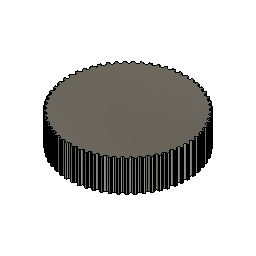
gear_61z (Autodesk Fusion 360 design; units mm, degrees)
Autodesk Fusion 360 part; units mm, degrees
sketch "Sketch1" plane through (0, 0, 0) normal (0, 0, 1) x (1, 0, 0) in component "gt2 pulley"
  circle A0 centre (0, 0) radius 19.4169 construction
  circle A1 centre (0, 0) radius 18.4129 construction
  line L0 (0, 0) -> (0, 19.4169) construction
  line L1 (0, 0) -> (0.9996, 19.3912) construction
  line L2 (0, 0) -> (1.4062, 19.3659) construction
  circle A2 centre (0, 0) radius 19.1629 construction
  arc A3 (0.3916, 19.0246) -> (0.4635, 18.7309) centre (1.3878, 19.1126) ccw
  circle A4 centre (0, 0) radius 19.0129 construction
  arc A5 (0.2441, 19.1613) -> (0, 19.1629) centre (0, 0) ccw
  arc A6 (0.3916, 19.0246) -> (0.2441, 19.1613) centre (0.2422, 19.0114) ccw
  arc A7 (0.4635, 18.7309) -> (0.9479, 18.3885) centre (0.9764, 18.9428) ccw
  arc A8 (0, 19.1629) -> (-0.2441, 19.1613) centre (0, 0) ccw
  arc A9 (-0.2441, 19.1613) -> (-0.3916, 19.0246) centre (-0.2422, 19.0114) ccw
  arc A10 (-0.4635, 18.7309) -> (-0.3916, 19.0246) centre (-1.3878, 19.1126) ccw
  arc A11 (-0.9479, 18.3885) -> (-0.4635, 18.7309) centre (-0.9764, 18.9427) ccw
  arc A12 (0.9479, 18.3885) -> (-0.9479, 18.3885) centre (0, 0) ccw
  point P0 (1.3878, 19.1126)
  point P1 (0, 19.1629)
  dimension "d18" = 38.8338
  dimension "d19" = 2.951
  dimension "d22" = 1.004
  dimension "d24" = 0.75
  dimension "d26" = 1
  dimension "d27" = 0.15
  dimension "d28" = 0.15
  dimension "d47" = 0.555
  dimension "d52" = 3.812
  constraint coincident A0.centre A1.centre
  constraint coincident A0 L0.end
  constraint vertical L0
  constraint coincident A0 L1.end
  constraint coincident A0 L2.end
  constraint concentric A1 A2
  constraint coincident A1 A7.end
  constraint coincident L1 A7.end
  constraint coincident A2 P0
  constraint coincident L2 P0
  constraint coincident P0 A3.centre
  constraint coincident A2 P1
  constraint coincident L0 P1
  constraint concentric A2 A4
  constraint coincident P1 A5.end
  constraint coincident A4 A6.centre
  constraint coincident A3.start A6.start
  constraint tangent A3 A6
  constraint tangent A3 A7
  constraint symmetric L0 A7.end A11.start
  constraint symmetric L0 A3.start A9.end
  constraint symmetric L0 A3.end A10.start
  constraint symmetric L0 A3 A10
  constraint symmetric L0 A5.start A8.end
  constraint symmetric L0 P1 A5.end
  constraint symmetric L0 A5 A8
  constraint symmetric L0 A6 A9
  constraint symmetric L0 A7 A11
  constraint coincident A1 A11.start
  constraint tangent A1 A7
  constraint coincident L1 A7.centre
  measures "d18" diameter of A0
  measures "d19" angle of L0 L1
  measures "d22" distance of A0 A1
  measures "d24" distance of A1 A2
  measures "d26" radius of A3
  measures "d27" distance of A2 A4
  measures "d28" radius of A6
  measures "d47" radius of A7
extrude "Extrude1" add sketch "Sketch1" along normal blind 10 makes body 1
pattern_circular "C-Pattern1" count 61 over 360 about axis through (0, 0, 1.75) along (0, 0, 1) of bodies 1 makes body 2 at (-2.6252, 18.2248, 6.6667) makes body 3 at (-3.8695, 18.0017, 6.6667) makes body 4 at (-6.2976, 17.3025, 6.6667) makes body 5 at (-6.6919, 17.1538, 3.3333) makes body 6 at (-9.1608, 15.9723, 6.6667) makes body 7 at (-10.0593, 15.4222, 3.3333) makes body 8 at (-12.6994, 13.3327, 6.6667) makes body 9 at (-13.0012, 13.0385, 6.6667) makes body 10 at (-14.273, 11.6326, 3.3333) makes body 11 at (-15.3934, 10.1034, 3.3333) makes body 12 at (-16.9758, 7.1314, 6.6667) makes body 13 at (-17.1346, 6.741, 3.3333) makes body 14 at (-17.7369, 4.9435, 3.3333) makes body 15 at (-18.2737, 2.2597, 6.6667) makes body 16 at (-18.411, -0.2634, 6.6667) makes body 17 at (-18.4002, -0.6847, 3.3333) makes body 18 at (-18.2322, -2.573, 3.3333) makes body 19 at (-17.4589, -5.85, 6.6667) makes body 20 at (-17.0163, -7.0341, 6.6667) makes body 21 at (-16.2029, -8.7465, 6.6667) makes body 22 at (-15.6761, -9.6589, 3.3333) makes body 23 at (-14.0712, -11.8759, 6.6667) makes body 24 at (-13.3689, -12.6612, 3.3333) makes body 25 at (-11.9962, -13.9687, 3.3333) makes body 26 at (-10.4964, -15.1282, 3.3333) makes body 27 at (-8.8853, -16.1272, 3.3333) makes body 28 at (-6.3965, -17.2661, 6.6667) makes body 29 at (-4.5873, -17.8323, 6.6667) makes body 30 at (-3.5599, -18.0655, 6.6667) makes body 31 at (-0.8426, -18.3936, 6.6667) makes body 32 at (0.2107, -18.4117, 3.3333) makes body 33 at (2.1027, -18.2924, 6.6667) makes body 34 at (5.3985, -17.6037, 6.6667) makes body 35 at (6.5937, -17.1918, 6.6667) makes body 36 at (8.3264, -16.4227, 6.6667) makes body 37 at (9.252, -15.9196, 3.3333) makes body 38 at (11.5096, -14.3723, 6.6667) makes body 39 at (12.3128, -13.6905, 3.3333) makes body 40 at (14.2062, -11.7141, 6.6667) makes body 41 at (15.6761, -9.6589, 6.6667) makes body 42 at (15.8931, -9.2976, 3.3333) makes body 43 at (16.7648, -7.6141, 3.3333) makes body 44 at (17.871, -4.434, 6.6667) makes body 45 at (18.1332, -3.1974, 6.6667) makes body 46 at (18.3658, -1.316, 6.6667) makes body 47 at (18.4092, 0.3687, 6.6667) makes body 48 at (18.3405, 1.631, 3.3333) makes body 49 at (17.8961, 4.3317, 6.6667) makes body 50 at (17.1346, 6.741, 6.6667) makes body 51 at (16.9758, 7.1314, 3.3333) makes body 52 at (15.3934, 10.1034, 6.6667) makes body 53 at (14.6639, 11.1358, 6.6667) makes body 54 at (13.4412, 12.5845, 6.6667) makes body 55 at (12.076, 13.8998, 6.6667) makes body 56 at (10.5828, 15.0678, 6.6667) makes body 57 at (8.9774, 16.0761, 6.6667) makes body 58 at (7.2769, 16.914, 6.6667) makes body 59 at (6.2976, 17.3025, 3.3333) makes body 60 at (3.6632, 18.0448, 6.6667) makes body 61 at (1.7884, 18.3258, 6.6667)
sketch "Sketch2" plane through (0, 0, 10) normal (0, 0, 1) x (-1, 0, 0)
  arc A0 (-9.7114, -16.3639) -> (-9.6503, -16.5556) centre (-9.5748, -16.426) ccw
  arc A1 (-9.6503, -16.5556) -> (-9.2255, -16.7961) centre (0, 0) ccw
  arc A2 (-9.2255, -16.7961) -> (-9.0297, -16.7497) centre (-9.1532, -16.6646) ccw
  arc A3 (-8.8226, -16.5295) -> (-9.0297, -16.7497) centre (-8.2061, -17.3169) ccw
  arc A4 (-8.2323, -16.4701) -> (-8.8225, -16.5295) centre (-8.4804, -16.9665) ccw
  arc A5 (-9.8821, -15.5364) -> (-8.2323, -16.4701) centre (0, 0) ccw
  arc A6 (-9.6292, -16.073) -> (-9.8821, -15.5364) centre (-10.18, -16.0047) ccw
  arc A7 (-9.7114, -16.3639) -> (-9.6292, -16.073) centre (-10.6216, -15.9499) ccw
  circle A8 centre (0, 0) radius 18.4129
  constraint coincident A1.centre A5.centre
extrude "Extrude2" add sketch "Sketch2" against normal blind 10 contours A5 A8 bodies 1 2 4 6 8 10 12 14 16 18 20 22 24 26 28 30 32 34 36 38 40 42 44 46 48 50 52 54 56 58 60
combine "Combine1" operation add target body 9 tool bodies 55 1 3 59 57 7 61 5 31 45 15 17 37 35 19 33 11 13 53 51 47 21 39 29 41 43 23 25 49 27
extrude "Extrude4" [suppressed] in component "gt2 pulley"
pattern_circular "C-Pattern7" [suppressed] in component "gt2 pulley"
extrude "Extrude3" [suppressed] in component "gt2 pulley"
pattern_circular "C-Pattern6" [suppressed] in component "gt2 pulley"
extrude "Extrude2'" [suppressed] in component "gt2 pulley"
pattern_circular "C-Pattern5" [suppressed] in component "gt2 pulley"
extrude "Extrude1'" [suppressed] in component "gt2 pulley"
pattern_circular "C-Pattern4" [suppressed] in component "gt2 pulley"
pattern_circular "C-Pattern3" [suppressed] in component "gt2 pulley"
pattern_circular "C-Pattern2" [suppressed] in component "gt2 pulley"
pattern_circular "C-Pattern1'" [suppressed] in component "gt2 pulley"
copy_body "Body->Comp1" [suppressed] in component "Component"
copy_body "Body->Comp2" [suppressed] in component "Component'"
copy_body "Body->Comp3" [suppressed] in component "Component''"
copy_body "Body->Comp4" [suppressed] in component "Component'''"
copy_body "Body->Comp5" [suppressed] in component "Component''''"
copy_body "Body->Comp6" [suppressed] in component "Component'''''"
copy_body "Body->Comp7" [suppressed] in component "Component''''''"
copy_body "Body->Comp8" [suppressed] in component "Component'''''''"
copy_body "Body->Comp9" [suppressed] in component "Component''''''''"
copy_body "Body->Comp10" [suppressed] in component "Component'''''''''"
copy_body "Body->Comp11" [suppressed] in component "Component''''''''''"
copy_body "Body->Comp12" [suppressed] in component "Component'''''''''''"
copy_body "Body->Comp13" [suppressed] in component "Component''''''''''''"
copy_body "Body->Comp14" [suppressed] in component "Component'''''''''''''"
copy_body "Body->Comp15" [suppressed] in component "Component''''''''''''''"
copy_body "Body->Comp16" [suppressed] in component "Component'''''''''''''''"
copy_body "Body->Comp17" [suppressed] in component "Component''''''''''''''''"
copy_body "Body->Comp18" [suppressed] in component "Component'''''''''''''''''"
copy_body "Body->Comp19" [suppressed] in component "Component''''''''''''''''''"
copy_body "Body->Comp20" [suppressed] in component "Component'''''''''''''''''''"
component "gt2 pulley" placed x (1, 0, 0) y (0, 1, 0) z (0, 0, 1) at (0, 0, 0)
equation "NumTeeth = 61" comment "min 20"
equation "ToothPitch = 2 mm"
equation "PullyDia = NumTeeth * ToothPitch / PI"
equation "ToothAng = ( ( 360 / NumTeeth ) * 1 deg )"
equation "TransOffsetAngle = ToothAng * 0.2"
equation "Sholulder_Radius = 0.15 mm"
equation "Root_Radius = 0.555 mm"
equation "TransRadius = 1 mm"
equation "ToolHeight = 0.75 mm"
equation "PLD = 0.254 mm"
equation "d18 = PullyDia"
equation "d19 = ToothAng / 2"
equation "d22 = PLD + ToolHeight"
equation "d24 = ToolHeight"
equation "d26 = TransRadius"
equation "d27 = Sholulder_Radius"
equation "d31 = NumTeeth"
equation "d33 = NumTeeth"
equation "d35 = NumTeeth"
equation "d37 = NumTeeth"
equation "d41 = NumTeeth"
equation "d45 = NumTeeth"
equation "d47 = Root_Radius"
equation "d50 = NumTeeth"
